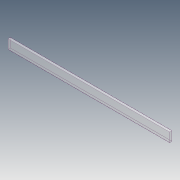
# Autodesk Inventor part: N/A
Saved by Autodesk Inventor 2015 SP1 (Build 190203100, 203)
## iProperties
Created: 2015-05-20
Material: ACRYLIC, CLEAR
Vendor: HHMI: JRC - ID&F
Document SubType Name: Modeling
Designer: ARNOLDJ
Density: 0.66 g/cm^3
Appearance: Polycarbonate (Clear)
Description: MBS TROUGH SIDE
Part Number: N/A
Project: P-201804
RuleStatus: InUse
AfterDocSave0: file://Part Number Cleaner
LAB/DEPT: SVOBODA (LAB)
REQUESTING SCIENTIST: SOFRONIEW, NICK
SURFACE ROUGHNESS: N/A
DESIGN DEPARTMENT: HHMI: JRC - ID&F
SPECIAL FINISH: NONE
ALTERED ITEM PART NUMBER: N/A
ALTERED ITEM VENDOR: N/A
ALTERED ITEM DESCRIPTION: N/A
Revision Number: -
Autodesk Inventor part; units mm, degrees
ref_plane "YZ Plane" through (0, 0, 0) normal (1, 0, 0) x (0, 1, 0)
ref_plane "XZ Plane" through (0, 0, 0) normal (0, 1, 0) x (-1, 0, 0)
ref_plane "XY Plane" through (0, 0, 0) normal (0, 0, 1) x (1, 0, 0)
sketch "Sketch1" plane through (0, 0, 0) normal (0, 0, 1) x (1, 0, 0)
  line L0 (0, 17.78) -> (0, -17.78) projected
  line L1 (-315.595, 0) -> (315.595, 0) projected
  line L2 (225.425, -12.7) -> (-225.425, -12.7)
  line L3 (-225.425, -12.7) -> (-225.425, 12.7)
  line L4 (-225.425, 12.7) -> (225.425, 12.7)
  line L5 (225.425, 12.7) -> (225.425, -12.7)
  line L6 (225.425, -12.7) -> (-225.425, 12.7) construction
  line L7 (-225.425, -12.7) -> (225.425, 12.7) construction
  point P0 (0, 0)
  dimension "d0" = 450.85
  dimension "d1" = 25.4
  constraints: 12 end point, 2 midpoint, 2 parallel, 1 horizontal, 1 perpendicular
  measures "d0" distance of L3.end L4.end
  measures "d1" distance of L2.end L3.end
extrude "Extrusion1" add sketch "Sketch1" along normal mid plane 6.35
body "Solid1"
